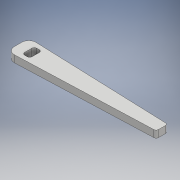
# Autodesk Inventor part: slider_link_p3
Saved by Autodesk Inventor 2017 (Build 210142000, 142)
## iProperties
Created: 2018-02-05
Part Number: slider_link_p3
Material: Generic
Document SubType Name: Modeling
Designer: Nic
Density: 1 g/cm^3
Appearance: Default
Author: Nic
Autodesk Inventor part; units mm, degrees
ref_plane "YZ Plane" through (0, 0, 0) normal (1, 0, 0) x (0, 1, 0)
ref_plane "XZ Plane" through (0, 0, 0) normal (0, 1, 0) x (-1, 0, 0)
ref_plane "XY Plane" through (0, 0, 0) normal (0, 0, 1) x (1, 0, 0)
sketch "Sketch1" plane through (0, 0, 0) normal (0, 0, 1) x (1, 0, 0)
  line L0 (-2.8894, 4.6352) -> (55.0041, 2.4993)
  line L1 (55.0041, -2.4993) -> (-2.8894, -4.6352)
  line L2 (-6, -1.6373) -> (-6, 1.6373)
  line L3 (-0.6, 2.6) -> (0.6, 2.6)
  line L4 (1.6, 1.6) -> (1.6, -1.6)
  line L5 (0.6, -2.6) -> (-0.6, -2.6)
  line L6 (-1.6, -1.6) -> (-1.6, 1.6)
  line L7 (0, 0) -> (0, 4.5286) construction
  line L8 (0, 0) -> (-6, 0) construction
  arc A0 (-2.8894, 4.6352) -> (-6, 1.6373) centre (-3, 1.6373) ccw
  arc A1 (-6, -1.6373) -> (-2.8894, -4.6352) centre (-3, -1.6373) ccw
  arc A2 (55.9672, 1.5) -> (55.0041, 2.4993) centre (54.9672, 1.5) ccw
  arc A3 (55.0041, -2.4993) -> (55.9672, -1.5) centre (54.9672, -1.5) ccw
  arc A4 (-0.6, 2.6) -> (-1.6, 1.6) centre (-0.6, 1.6) ccw
  arc A5 (1.6, 1.6) -> (0.6, 2.6) centre (0.6, 1.6) ccw
  arc A6 (0.6, -2.6) -> (1.6, -1.6) centre (0.6, -1.6) ccw
  arc A7 (-1.6, -1.6) -> (-0.6, -2.6) centre (-0.6, -1.6) ccw
  line L9 (55.9672, 1.5) -> (55.9672, -1.5)
  point P0 (-6, 4.75)
  point P1 (-6, -4.75)
  point P2 (-1.6, 2.6)
  point P3 (1.6, -2.6)
  point P4 (1.6, 2.6)
  dimension "d0" = 6
  dimension "d2" = 3.2
  dimension "d3" = 5.2
  dimension "d4" = 9.5
  dimension "d5" = 3
  dimension "d6" = 3
  dimension "d7" = 1
  dimension "d8" = 1
  dimension "d9" = 3
  dimension "d14" = 3.2746
  constraints: 20 end point, 16 point on circle, 16 tangent, 11 point on line, 8 centre point, 4 equal radius, 2 parallel, 2 perpendicular, 1 horizontal, 1 midpoint, 1 vertical, 3 other
  measures "d0" distance from line of L7.start L2
  measures "d2" distance of point (-1.6, 2.6) point (1.6, 2.6)
  measures "d3" distance of point (1.6, 2.6) point (1.6, -2.6)
  measures "d4" distance of point (-6, -4.75) point (-6, 4.75)
  measures "d5" radius of A0
  measures "d6" radius of A1
  measures "d7" radius of A2
  measures "d8" radius of A4
  measures "d9" distance of L9.start L9.end
  measures "d14" distance of L2.start L2.end
extrude "Extrusion1" add sketch "Sketch1" along normal blind 3
body "Solid1"
